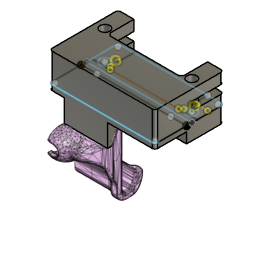
chase_mount (Autodesk Fusion 360 design; units mm, degrees)
Autodesk Fusion 360 part; units mm, degrees
note: some values were not read from the file. Set by a fixed rule: which sketch regions a step uses.
sketch "Sketch1" plane through (0, 0, 0) normal (0, 0, 1) x (1, 0, 0)
  line L0 (-15, 10) -> (-20, 10)
  line L1 (-20, 9) -> (-20, 1)
  line L2 (20, 1) -> (20, 10)
  line L3 (-19, 10) -> (-16.5, 10) construction
  line L4 (-16.5, 10) -> (-16.5, 6.5) construction
  line L5 (-16.5, 6.5) -> (-20, 6.5) construction
  line L6 (-20, 6.5) -> (-20, 10) construction
  line L7 (20, 10) -> (16.5, 10) construction
  line L8 (16.5, 10) -> (16.5, 6.5) construction
  line L9 (16.5, 6.5) -> (20, 6.5) construction
  line L10 (20, 6.5) -> (20, 9) construction
  circle A0 centre (-16.5, 6.5) radius 1.7
  circle A1 centre (16.5, 6.5) radius 1.7
  arc A2 (-19, 10) -> (-20, 9) centre (-19, 9) ccw
  arc A3 (20, 9) -> (19, 10) centre (19, 9) ccw
  line L11 (13, 5) -> (-13, 5)
  line L12 (-14, 6) -> (-14, 9)
  line L13 (14, 9) -> (14, 6)
  arc A4 (-14, 9) -> (-15, 10) centre (-15, 9) ccw
  line L14 (19, 10) -> (15, 10)
  arc A5 (15, 10) -> (14, 9) centre (15, 9) ccw
  line L15 (-14, 6) -> (-13, 5)
  line L16 (13, 5) -> (14, 6)
  line L17 (-19, 0) -> (19, 0)
  line L18 (20, 10) -> (0, 0) construction
  line L19 (-20, 10) -> (0, 0) construction
  arc A6 (-20, 1) -> (-19, 0) centre (-19, 1) ccw
  arc A7 (19, 0) -> (20, 1) centre (19, 1) ccw
  point P0 (14, 5)
  point P1 (-14, 5)
  dimension "d3" = 3.5
  dimension "d4" = 3.5
  dimension "d5" = 3.5
  dimension "d6" = 3.5
  dimension "d7" = 3.4
  dimension "d8" = 3.4
  dimension "d9" = 1
  dimension "d32" = 1
  dimension "d33" = 1
  dimension "d34" = 1
  dimension "d35" = 1
  dimension "d36" = 1
  dimension "d37" = 1
  dimension "d44" = 1
  constraint horizontal L0
  constraint perpendicular L0 L1
  constraint parallel L1 L2
  constraint coincident L19.end L18
  constraint coincident L18.end L19
  constraint coincident L18.end L19.end
  constraint horizontal L3
  constraint vertical L4
  constraint horizontal L5
  constraint vertical L6
  constraint horizontal L7
  constraint vertical L8
  constraint horizontal L9
  constraint vertical L10
  constraint coincident L4.end L5.start
  constraint coincident L8.end L9.start
  constraint coincident L0.end L3
  constraint coincident L0.end L1
  constraint tangent L3 A2
  constraint tangent L1 A2
  constraint coincident L2.end L0
  constraint coincident L2.end L10
  constraint tangent L0 A3
  constraint tangent L10 A3
  constraint equal A2 A3
  constraint horizontal L11
  constraint perpendicular L11 L12
  constraint parallel L12 L13
  constraint coincident L0 A3.end
  constraint tangent L0 A4
  constraint tangent L12 A4
  constraint tangent L13 A5
  constraint tangent L14 A5
  constraint coincident P1 L12
  constraint coincident P1 L11
  constraint coincident P0 L11
  constraint coincident P0 L13
  constraint perpendicular L2 L17
  constraint coincident L17 L18.end
  constraint tangent L1 A6
  constraint tangent L17 A6
  constraint tangent L17 A7
  constraint tangent L2 A7
  constraint equal A6 A7
  measures "d3" distance of L0.end L3.end
  measures "d4" distance of L0.end L5.end
  measures "d5" distance of L2.end L7.end
  measures "d6" distance of L2.end L9.end
  measures "d7" diameter of A0
  measures "d8" diameter of A1
  measures "d9" radius of A2
  measures "d32" radius of A4
  measures "d33" radius of A5
  measures "d34" distance of P1 L12.start
  measures "d35" distance of P1 L11.end
  measures "d36" distance of P0 L11.start
  measures "d37" distance of P0 L13.end
  measures "d44" radius of A6
extrude "Extrude2" [suppressed]
sketch "Sketch2" plane through (0, 0, 3) normal (0, 0, 1) x (-1, 0, 0)
  line L0 (-20, -1) -> (-20, -9)
  arc A0 (-20, -9) -> (-19, -10) centre (-19, -9) ccw
  line L1 (15, -10) -> (19, -10)
  arc A1 (19, -10) -> (20, -9) centre (19, -9) ccw
  line L2 (20, -9) -> (20, -1)
  line L3 (19, -15) -> (-19, -15)
  line L4 (-20, -14) -> (-20, -5)
  line L5 (20, -5) -> (20, -14)
  arc A2 (19, -15) -> (20, -14) centre (19, -14) ccw
  arc A3 (-20, -14) -> (-19, -15) centre (-19, -14) ccw
  circle A4 centre (16.5, -6.5) radius 1.875
  circle A5 centre (-16.5, -6.5) radius 1.875
  line L6 (14, 11) -> (-14, 11)
  line L7 (20, -5) -> (-20, -5)
  line L8 (14, -6) -> (14, -9)
  arc A6 (14, -9) -> (15, -10) centre (15, -9) ccw
  line L9 (-19, -10) -> (-15, -10)
  arc A7 (-15, -10) -> (-14, -9) centre (-15, -9) ccw
  line L10 (-14, -9) -> (-14, -6)
  line L11 (-14, -6) -> (-13, -5)
  line L12 (-13, -5) -> (13, -5)
  line L13 (13, -5) -> (14, -6)
  line L14 (14, 11) -> (19, 11)
  line L15 (20, 10) -> (20, -1)
  line L16 (-14, 11) -> (-19, 11)
  line L17 (-20, 10) -> (-20, -1)
  arc A8 (20, 10) -> (19, 11) centre (19, 10) ccw
  arc A9 (-19, 11) -> (-20, 10) centre (-19, 10) ccw
  line L18 (20, -1) -> (20, -3)
  line L19 (-20, -3) -> (-20, -1)
  line L20 (-20, -1) -> (20, -1)
  line L21 (-20, -5) -> (-20, -3)
  line L22 (20, -3) -> (-20, -3)
  line L23 (20, -5) -> (20, -3)
  line L24 (-14, -9) -> (-14, -15)
  line L25 (14, -8.4776) -> (14, -15)
  point P0 (-14, -1)
  point P1 (14, -1)
  dimension "d14" = 1
  dimension "d15" = 3.75
  dimension "d16" = 3.75
  dimension "d24" = 28
  dimension "d49" = 1
  constraint horizontal L3
  constraint vertical L4
  constraint vertical L5
  constraint midpoint L0 L4.end
  constraint tangent L3 A2
  constraint tangent L5 A2
  constraint tangent L3 A3
  constraint tangent L4 A3
  constraint equal A2 A3
  constraint perpendicular L0 L7
  constraint horizontal L14
  constraint vertical L15
  constraint coincident L2.end L15.end
  constraint horizontal L16
  constraint vertical L17
  constraint coincident L0.start L17.end
  constraint tangent L15 A8
  constraint tangent L14 A8
  constraint tangent L16 A9
  constraint tangent L17 A9
  constraint equal A8 A9
  constraint coincident L2 L18.end
  constraint perpendicular L7 L18
  constraint coincident L0 L19.start
  constraint perpendicular L7 L21
  constraint perpendicular L21 L22
  constraint coincident A7.end L10.start
  constraint tangent A7 L24
  constraint coincident L8 L25.start
  constraint coincident L3 L25.end
  constraint perpendicular L3 L25
  measures "d14" radius of A2
  measures "d15" diameter of A4
  measures "d16" diameter of A5
  measures "d24" distance of L6.start L6.end
  measures "d49" radius of A8
extrude "Extrude3" add sketch "Sketch2" along normal blind 11 and the other way blind -7 contours L0 L2 L18 L19 L20 L22 | L0 L2 A4 A5 L7 L12 L21 L22 L23 | L0 A0 L4 A5 L7 L9 A7 L10 L11 | A0 L3 L4 A3 L9 A7 L24 | L1 A1 L2 L5 A4 L7 L8 A6 L13 L25 | L1 A1 L3 L5 A2 A6 L25 makes body 1
other "Base Mesh Feature2"
other "Scale1"
other "Modify1"
other "Modify2"
other "Modify3"
extrude "Extrude5" add sketch "Sketch2" against normal blind 2 contours L6 L14 L15 L16 L17 A8 A9 L20 makes body 2
other "Modify4"
sketch "Sketch5" plane through (-20, 0, 0) normal (-1, 0, 0) x (0, -1, 0)
  line L0 (-1, 1) -> (10, 1)
  line L1 (10, 1) -> (10, 3)
  line L2 (10, 3) -> (-1, 3)
  line L3 (6.1406, 1) -> (6.1406, -3.7684)
  line L4 (6.1406, -3.7684) -> (9, -7.5)
  line L5 (9, -7.5) -> (11, -7.5)
  line L6 (11, -7.5) -> (11, 1)
  line L7 (11, 1) -> (6.1406, 1)
  line L8 (0, 1) -> (1.1368, 1)
  line L9 (0, -1) -> (0, 1)
  line L10 (1.1368, 1) -> (0, -1)
  line L11 (-1, 3) -> (-1, 1)
  constraint coincident L0 L3.start
  constraint perpendicular L0 L3
  constraint perpendicular L3 L5
  constraint perpendicular L0 L6
  constraint perpendicular L3 L7
  constraint coincident L0 L8.start
  constraint coincident L0 L8.end
  constraint perpendicular L8 L9
extrude "Extrude7" add sketch "Sketch5" along normal blind -22 and the other way blind 5.6 contours L0 L8 L9 L10 | L0 L3 L4 L5 L6 L7 bodies 2
extrude "Extrude8" add sketch "Sketch2" along normal blind 11 contours L6 L14 L15 L16 L17 A8 A9 L20 bodies 1 2
extrude "Extrude9" add sketch "Sketch2" along normal blind 7 and the other way blind 6 contours L0 L2 L18 L19 L20 L22 bodies 1
extrude "Extrude10" add sketch "Sketch2" along normal blind 3.8 and the other way blind 6 contours L0 L2 A4 A5 L7 L12 L21 L22 L23 | L0 A0 L4 A5 L7 L9 A7 L10 L11 | A0 L3 L4 A3 L9 A7 L24 | L1 A1 L2 L5 A4 L7 L8 A6 L13 L25 | L1 A1 L3 L5 A2 A6 L25 bodies 1
other "Scale2"
other "Modify5"
equation "d35 = d34"
equation "d37 = d36"
